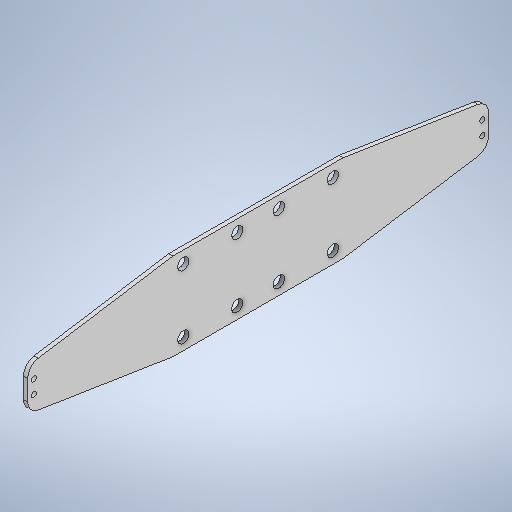
# Autodesk Inventor part: ENDSTOPPLATE_XAXIS
Saved by Autodesk Inventor 2025.2 (Build 292293000, 293)
## iProperties
Created: 2026-03-18
Part Number: ENDSTOPPLATE_XAXIS
Material: Generic
Document SubType Name: Modeling
Designer: composite
Density: 1 g/cm^3
Appearance: Default
Author: composite
Autodesk Inventor part; units mm, degrees
ref_plane "YZ Plane" through (0, 0, 0) normal (1, 0, 0) x (0, 1, 0)
ref_plane "XZ Plane" through (0, 0, 0) normal (0, 1, 0) x (-1, 0, 0)
ref_plane "XY Plane" through (0, 0, 0) normal (0, 0, 1) x (1, 0, 0)
sketch "Sketch1" plane through (0, 0, 0) normal (1, 0, 0) x (0, 1, 0)
  circle A0 centre (0, 0) radius 2.75
  line L0 (0, 0) -> (0, -10) construction
  line L1 (0, 0) -> (-10, 0) construction
  circle A1 centre (0, -26) radius 2.75
  circle A2 centre (-30.5, 0) radius 2.75
  circle A3 centre (-30.5, -26) radius 2.75
  circle A4 centre (0, -46) radius 2.75
  line L2 (0, -46) -> (0, -56) construction
  line L3 (0, -46) -> (-10, -46) construction
  circle A5 centre (0, -72) radius 2.75
  circle A6 centre (-30.5, -46) radius 2.75
  circle A7 centre (-30.5, -72) radius 2.75
  line L4 (5.75, 5) -> (-36.25, 5)
  line L5 (-36.25, 5) -> (-36.25, -77)
  line L6 (-36.25, -77) -> (5.75, -77)
  line L7 (5.75, -77) -> (5.75, 5)
  line L8 (5.75, -77) -> (-4.4535, -141.9314)
  line L9 (-10.3808, -147) -> (-20.1192, -147)
  line L10 (-26.0465, -141.9314) -> (-36.25, -77)
  circle A8 centre (-12, -144) radius 1.25
  circle A9 centre (-18.5, -144) radius 1.25
  line L11 (-12, -144) -> (-18.5, -144) construction
  line L12 (5.75, -36) -> (-36.25, -36) construction
  line L13 (5.75, 5) -> (-4.4535, 69.9314)
  line L14 (-10.3808, 75) -> (-20.1192, 75)
  line L15 (-26.0465, 69.9314) -> (-36.25, 5)
  circle A10 centre (-12, 72) radius 1.25
  circle A11 centre (-18.5, 72) radius 1.25
  line L16 (-12, 72) -> (-18.5, 72) construction
  arc A12 (-10.3808, -147) -> (-4.4535, -141.9314) centre (-10.3808, -141) ccw
  arc A13 (-26.0465, -141.9314) -> (-20.1192, -147) centre (-20.1192, -141) ccw
  arc A14 (-4.4535, 69.9314) -> (-10.3808, 75) centre (-10.3808, 69) ccw
  arc A15 (-20.1192, 75) -> (-26.0465, 69.9314) centre (-20.1192, 69) ccw
  point P0 (-5.25, -147)
  point P1 (-25.25, -147)
  point P2 (-15.25, -147)
  point P3 (-15.25, -77)
  point P4 (-15.25, -144)
  point P5 (-5.25, 75)
  point P6 (-25.25, 75)
  point P7 (-15.25, 75)
  point P8 (-15.25, 72)
  dimension "d0" = 5.5
  dimension "d1" = 10
  dimension "d2" = 10
  dimension "d5" = 26
  dimension "d8" = 30.5
  dimension "d13" = 46
  dimension "d18" = 5
  dimension "d19" = 5
  dimension "d20" = 5.75
  dimension "d21" = 5.75
  dimension "d22" = 70
  dimension "d23" = 20
  dimension "d24" = 2.5
  dimension "d25" = 2.5
  dimension "d26" = 3
  dimension "d27" = 6.5
  dimension "d28" = 6
  constraints: 34 end point, 16 centre point, 8 point on circle, 8 point on line, 8 tangent, 6 symmetric about line, 5 horizontal, 5 midpoint, 3 equal radius, 3 vertical, 2 coincident, 2 parallel, 2 vertical alignment, 1 collinear, 1 horizontal alignment, 1 perpendicular, 20 other
  measures "d0" diameter of A0
  measures "d1" distance of L0.start L0.end
  measures "d2" distance of L0.start L1.end
  measures "d5" distance of L0.start A1.centre
  measures "d8" distance of L0.start A2.centre
  measures "d13" distance of point (0, 0) point (0, -46)
  measures "d18" distance from line of L6 A5.centre
  measures "d19" distance from line of L0.start L4
  measures "d20" distance from line of L0.start L7
  measures "d21" distance from line of L5 A2.centre
  measures "d22" distance between parallel lines of L9 L6
  measures "d23" distance of point (-5.25, -147) point (-25.25, -147)
  measures "d24" diameter of A8
  measures "d25" diameter of A9
  measures "d26" distance from line of L9 L11.start
  measures "d27" distance of L11.end L11.start
  measures "d28" radius of A12
extrude "Extrusion1" add sketch "Sketch1" along normal blind 2
equation "\"d18\" = d19"
equation "\"d21\" = d20"
equation "\"d25\" = d24"
body "Solid1"
